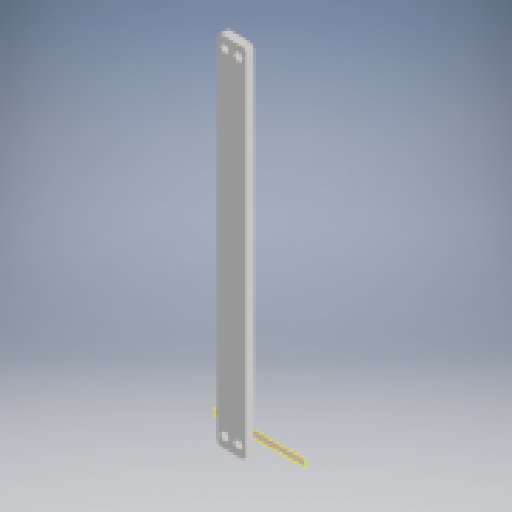
# Autodesk Inventor part: Schroff_Back_Stabilizer
Saved by Autodesk Inventor 2025.2 (Build 292293000, 293)
## iProperties
Created: 2024-12-11
Part Number: Schroff_Back_Stabilizer
Material: Generic
Document SubType Name: Modeling
Designer: Paul Linke
Density: 1 g/cm^3
Appearance: Default
Author: Paul Linke
Autodesk Inventor part; units mm, degrees
ref_plane "YZ Plane" through (0, 0, 0) normal (1, 0, 0) x (0, 1, 0)
ref_plane "XZ Plane" through (0, 0, 0) normal (0, 1, 0) x (-1, 0, 0)
ref_plane "XY Plane" through (0, 0, 0) normal (0, 0, 1) x (1, 0, 0)
ref_plane "Work Plane1" through (0, 0, 0) normal (0, 0, 1) x (1, 0, 0)
sketch "Sketch1" plane through (0, 0, 0) normal (0, 0, 1) x (1, 0, 0)
  line L0 (-31, 2.95) -> (-31, 4.9) projected
  line L1 (-31, 0) -> (-1, 0) projected
  line L2 (-1, 130.25) -> (-31, 130.25) projected
  line L3 (-1, 130.05) -> (-1, 128.3) projected
  line L4 (-1, 0.2) -> (-1, 1.95) projected
  line L5 (-28.5104, 0) -> (-18.3504, 0)
  line L6 (-18.3504, 0) -> (-18.3504, 130.25)
  line L7 (-18.3504, 130.25) -> (-28.5104, 130.25)
  line L8 (-28.5104, 130.25) -> (-28.5104, 0)
  line L9 (-28.5104, 3.925) -> (-18.3504, 3.925) construction
  line L10 (-28.5104, 126.325) -> (-18.3504, 126.325) construction
  circle A0 centre (-25.9704, 3.925) radius 1.45
  circle A1 centre (-20.8904, 3.925) radius 1.45
  line L11 (-23.4304, 3.925) -> (-23.4304, 126.325) construction
  line L12 (-23.4304, 126.325) -> (-23.4304, 248.725) construction
  circle A2 centre (-25.9704, 126.325) radius 1.45
  circle A3 centre (-20.8904, 126.325) radius 1.45
  point P0 (0, 0)
  dimension "d0" = 10.16
  dimension "d1" = 3.925
  dimension "d2" = 3.925
  dimension "d3" = 2.9
  dimension "d4" = 2.9
  dimension "d5" = 2.54
  dimension "d6" = 2.54
  dimension "d9" = 122.4
  constraints: 16 end point, 8 point on line, 4 centre point, 3 perpendicular, 2 midpoint, 2 parallel, 1 collinear, 1 horizontal, 1 vertical, 6 other
  measures "d0" distance between parallel lines of L6 L8
  measures "d1" distance between parallel lines of L1 L9
  measures "d2" distance between parallel lines of L2 L10
  measures "d3" diameter of A0
  measures "d4" diameter of A1
  measures "d5" distance from line of A0.centre L8
  measures "d6" distance from line of L6 A1.centre
  measures "d9" distance of L11.start L12.start
extrude "Extrusion1" add sketch "Sketch1" along normal blind 3
fillet "Fillet1" radius 1.5 4 edges at (-28.5104, 0, 1.5) (-28.5104, 130.25, 1.5) (-18.3504, 130.25, 1.5) (-18.3504, 0, 1.5)
body "Solid1"
